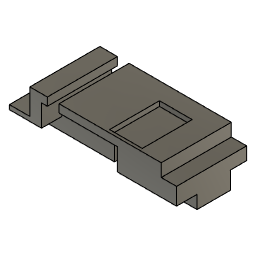
gc power usb c bracket (Autodesk Fusion 360 design; units mm, degrees)
Autodesk Fusion 360 part; units mm, degrees
sketch "Sketch1" plane through (0, 0, 0) normal (0, 1, 0) x (1, 0, 0)
  line L0 (0, 0) -> (25, 0)
  line L1 (25, 0) -> (25, -7)
  line L2 (25, -7) -> (1, -7)
  line L3 (0, -5) -> (0, 0)
  line L4 (-5, 5) -> (30, 5)
  line L5 (30, 5) -> (30, -10)
  line L6 (30, -10) -> (-5, -10)
  line L7 (-5, -10) -> (-5, 5)
  line L8 (1, -7) -> (1, -10)
  line L9 (-1, -5) -> (-1, -10)
  line L10 (0, -5) -> (-1, -5)
  dimension "d1" = 25
  dimension "d2" = 5
  dimension "d4" = 6
  dimension "d5" = 2
  constraint horizontal L0
  constraint vertical L1
  constraint horizontal L2
  constraint vertical L3
  constraint coincident L0.start L3.end
  constraint coincident L6 L8.end
  constraint perpendicular L6 L8
  constraint coincident L6 L9.end
  constraint perpendicular L6 L9
  constraint parallel L0 L4
  constraint parallel L1 L5
  constraint parallel L2 L6
  constraint parallel L3 L7
  measures "d1" distance of L0.start L0.end
  measures "d2" distance of L0.start L3.start
  measures "d4" distance of L7 L8
  measures "d5" distance of L8 L9
extrude "Extrude1" add sketch "Sketch1" along normal blind 18 contours L0 L1 L2 L3 L4 L5 L6 L7 L8 L9 L10 makes body 1
move_face "OffsetFaces1" offset -1 1 faces at (0, 6, 3.3333) on bodies 1
move_face "OffsetFaces2" offset 2 2 faces at (20.3333, 6, 10) (-2.3333, 6, 10) on bodies 1
extrude "Extrude2" cut 1 faces at (1, 6, 8.6667) along direction (1, 0, 0) blind 4 on bodies 1 bodies 1
split "Split1" by plane through (-1, 0, 5) normal (1, 0, 0) bodies 1 makes body 2 at (19.6667, 12, -5)
sketch "Sketch3" plane through (-1, 0, 0) normal (1, 0, 0) x (0, 1, 0)
  line L0 (18, -5) -> (18, 12)
  line L1 (18, 12) -> (0, 12)
  line L2 (0, 12) -> (0, -5)
  line L3 (0, -5) -> (18, -5)
  line L4 (18, 12) -> (0, 12)
  line L5 (0, 12) -> (0, 7)
  line L6 (0, 7) -> (18, 7)
  line L7 (18, 7) -> (18, 12)
  constraint horizontal L4
  constraint vertical L5
  constraint horizontal L6
  constraint vertical L7
extrude "Extrude3" add sketch "Sketch3" along normal blind 2 contours L0 L1 L2 L4 L5 L6 L7 bodies 1
combine "Combine1" operation add target body 1 tool bodies 2
sketch "Sketch4" plane through (0, 0, 0) normal (0, -1, 0) x (1, 0, 0)
  line L0 (1, 12) -> (-5, 12)
  line L1 (-5, 12) -> (-5, -5)
  line L2 (-5, -5) -> (30, -5)
  line L3 (30, -5) -> (30, 12)
  line L4 (30, 12) -> (5, 12)
  line L5 (5, 12) -> (5, 7)
  line L6 (5, 7) -> (25, 7)
  line L7 (25, 7) -> (25, 0)
  line L8 (25, 0) -> (-1, 0)
  line L9 (-1, 0) -> (-1, 7)
  line L10 (-1, 7) -> (1, 7)
  line L11 (1, 7) -> (1, 12)
  line L12 (23, -5) -> (23, 0)
  line L13 (17, -5) -> (17, 0)
  dimension "d14" = 7
  dimension "d15" = 6
  constraint coincident L2 L12.start
  constraint coincident L8 L12.end
  constraint perpendicular L8 L12
  constraint coincident L2 L13.start
  constraint coincident L8 L13.end
  constraint perpendicular L8 L13
  measures "d14" distance of L3 L12
  measures "d15" distance of L12 L13
extrude "Extrude4" cut sketch "Sketch4" against normal blind 9 contours L2 L8 L12 L13 bodies 1
sketch "Sketch5" plane through (0, 18, 0) normal (0, 1, 0) x (-1, 0, 0)
  line L0 (-30, -5) -> (5, -5)
  line L1 (5, -5) -> (5, 12)
  line L2 (5, 12) -> (-1, 12)
  line L3 (-1, 12) -> (-1, 7)
  line L4 (-1, 7) -> (1, 7)
  line L5 (1, 7) -> (1, 0)
  line L6 (1, 0) -> (-25, 0)
  line L7 (-25, 0) -> (-25, 7)
  line L8 (-25, 7) -> (-5, 7)
  line L9 (-5, 7) -> (-5, 12)
  line L10 (-5, 12) -> (-30, 12)
  line L11 (-30, 12) -> (-30, -5)
  line L12 (-30, 1) -> (5, 1)
  dimension "d18" = 6
  constraint coincident L11 L12.start
  constraint coincident L1 L12.end
  constraint perpendicular L1 L12
  measures "d18" distance of L0 L12
extrude "Extrude5" cut sketch "Sketch5" against normal blind 6 contours L0 L1 L5 L6 L7 L11 L12 bodies 1
sketch "Sketch6" plane through (0, 0, 0) normal (0, -1, 0) x (1, 0, 0)
  line L0 (17, -5) -> (17, 0)
  line L1 (17, 0) -> (-1, 0)
  line L2 (-1, 0) -> (-1, 7)
  line L3 (-1, 7) -> (1, 7)
  line L4 (1, 7) -> (1, 12)
  line L5 (1, 12) -> (-5, 12)
  line L6 (-5, 12) -> (-5, -5)
  line L7 (-5, -5) -> (17, -5)
  line L8 (30, -5) -> (-5, -5)
  line L9 (-5, -5) -> (-5, 1)
  line L10 (-5, 1) -> (-1, 1)
  line L11 (-1, 1) -> (-1, 0)
  line L12 (-1, 0) -> (25, 0)
  line L13 (25, 0) -> (25, 1)
  line L14 (25, 1) -> (30, 1)
  line L15 (30, 1) -> (30, -5)
extrude "Extrude6" cut sketch "Sketch6" against normal blind 6 contours L0 L1 L2 L6 L7 L8 L9 L10 L11 L12 | L0 L8 L12 L13 L14 L15 bodies 1
extrude "Extrude7" add 2 faces at (20, 0, 10.3333) (-3.6667, 0, 6.6667) along direction (0, -1, 0) blind 6 on bodies 1 bodies 1
extrude "Extrude8" add 2 faces at (26, 6, -3.3333) (3.6667, 6, -3.3333) along direction (0, -1, 0) blind 5 on bodies 1 bodies 1
extrude "Extrude9" add 1 faces at (5, 7.3333, 0) along direction (0, 0, 1) blind 0.2 on bodies 1 bodies 1
extrude "Extrude10" add 2 faces at (-3.6667, -3.6667, 1) (26.6667, -3.6667, 1) along direction (0, 0, -1) blind 3 on bodies 1 bodies 1
extrude "Extrude11" add 1 faces at (5, 7.3333, 0.2) along direction (0, 0, 1) blind 0.5 on bodies 1 bodies 1
extrude "Extrude12" cut 2 faces at (26.6667, -3.6667, -2) (-3.6667, -3.6667, -2) along direction (0, 0, 1) blind 1 on bodies 1 bodies 1
extrude "Extrude13" add 1 faces at (30, 8, 8.3333) along direction (1, 0, 0) blind 10 on bodies 1 bodies 1
sketch "Sketch7" plane through (0, 0, 12) normal (0, 0, 1) x (-1, 0, 0)
  line L0 (-5, -18) -> (-5, 6)
  line L1 (-5, 6) -> (-40, 6)
  line L2 (-40, 6) -> (-40, -18)
  line L3 (-40, -18) -> (-5, -18)
  line L4 (-32.5, 5) -> (-32.5, -12.1)
  line L5 (-32.5, -12.1) -> (-21.3, -12.1)
  line L6 (-21.3, -12.1) -> (-21.3, 5)
  line L7 (-21.3, 5) -> (-32.5, 5)
  dimension "d40" = 11.2
  dimension "d41" = 17.1
  dimension "d42" = 7.5
  dimension "d43" = 1
  constraint horizontal L7
  constraint vertical L4
  constraint horizontal L5
  constraint vertical L6
  measures "d40" distance of L4.start L6.end
  measures "d41" distance of L5.end L6.end
  measures "d42" distance of L2 L4
  measures "d43" distance of L1 L7
extrude "Extrude14" cut sketch "Sketch7" against normal blind 0.7 contours L4 L5 L6 L7 bodies 1
extrude "Extrude15" cut 2 faces at (10.4333, 8.0333, 12) (-1, 2, 12) along direction (0, 0, -1) blind 1 on bodies 1 bodies 1
extrude "Extrude16" cut 1 faces at (25.0333, 0.7, 11.3) along direction (0, 0, -1) blind 1 on bodies 1 bodies 1
extrude "Extrude17" cut 2 faces at (10.4333, 8.0333, 11) (-1, 2, 11) along direction (0, 0, -1) blind 1.25 on bodies 1 bodies 1
extrude "Extrude18" cut 1 faces at (25.0333, 0.7, 10.3) along direction (0, 0, -1) blind 1.25 on bodies 1 bodies 1
extrude "Extrude19" add 1 faces at (20, 12, -3.1) along direction (0, 1, 0) blind 0.5 on bodies 1 bodies 1
extrude "Extrude20" cut 2 faces at (35, -3.6667, -1) (-3.6667, -3.6667, -1) along direction (0, 0, 1) blind 0.5 on bodies 1 bodies 1
sketch "Sketch8" plane through (40, 0, 0) normal (1, 0, 0) x (0, 1, 0)
  line L0 (1, -0.5) -> (1, -5)
  line L1 (1, -5) -> (12.5, -5)
  line L2 (12.5, -5) -> (12.5, 1)
  line L3 (12.5, 1) -> (18, 1)
  line L4 (18, 1) -> (18, 9.75)
  line L5 (18, 9.75) -> (-6, 9.75)
  line L6 (-6, 9.75) -> (-6, -0.5)
  line L7 (-6, -0.5) -> (1, -0.5)
  line L8 (18, 5.375) -> (-6, 5.375)
  constraint midpoint L4 L8.start
  constraint coincident L6 L8.end
  constraint perpendicular L6 L8
extrude "Extrude21" add sketch "Sketch8" along normal blind 22 contours L0 L1 L2 L3 L4 L6 L7 L8 bodies 1
extrude "Extrude22" cut 1 faces at (25.0333, 0.7, 9.05) along direction (0, 0, -1) blind 1 on bodies 1 bodies 1
extrude "Extrude23" cut 1 faces at (62, 8.6667, -1.5) along direction (-1, 0, 0) blind 8 on bodies 1 bodies 1
sketch "Sketch9" plane through (-5, 0, 0) normal (-1, 0, 0) x (0, -1, 0)
  line L0 (-1, -5) -> (-1, -0.5)
  line L1 (-1, -0.5) -> (6, -0.5)
  line L2 (6, -0.5) -> (6, 9.75)
  line L3 (6, 9.75) -> (-18, 9.75)
  line L4 (-18, 9.75) -> (-18, 1)
  line L5 (-18, 1) -> (-12.5, 1)
  line L6 (-12.5, 1) -> (-12.5, -5)
  line L7 (-12.5, -5) -> (-1, -5)
  line L8 (-12.5, 1) -> (6, 1)
  constraint coincident L5.end L6.start
  constraint coincident L2 L8.end
  constraint perpendicular L2 L8
extrude "Extrude24" add sketch "Sketch9" along normal blind 5 contours L0 L1 L2 L6 L7 L8 bodies 1
extrude "Extrude25" add 1 faces at (23, 12.5, -3.1) along direction (0, 1, 0) blind 1 on bodies 1 bodies 1
extrude "Extrude26" cut 1 faces at (54, 9.3333, -1.5) along direction (-1, 0, 0) blind 2.5 on bodies 1 bodies 1
extrude "Extrude27" cut 1 faces at (51.5, 9.3333, -1.5) along direction (-1, 0, 0) blind 0.5 on bodies 1 bodies 1
extrude "Extrude28" cut 1 faces at (22, 13.5, -3.1) along direction (0, -1, 0) blind 1 on bodies 1 bodies 1
extrude "Extrude29" cut 1 faces at (51, 8.6667, -1.5) along direction (-1, 0, 0) blind 5.75 on bodies 1 bodies 1
extrude "Extrude30" add 1 faces at (-10, 8.6667, -1.5) along direction (-1, 0, 0) blind 2 on bodies 1 bodies 1
equation "d40 = 10.70 mm + 0.5 mm"
equation "d41 = 16.20 mm + 0.9 mm"
